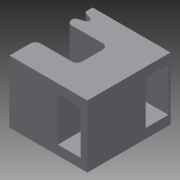
# Autodesk Inventor part: Hook2
Saved by Autodesk Inventor 2015 (Build 190159000, 159)
## iProperties
Created: 2015-01-19
Part Number: Hook2
Material: Generic
Document SubType Name: Modeling
Designer: nilesstanton
Density: 1 g/cm^3
Appearance: Default
Author: nilesstanton
Autodesk Inventor part; units mm, degrees
ref_plane "YZ Plane" through (0, 0, 0) normal (1, 0, 0) x (0, 1, 0)
ref_plane "XZ Plane" through (0, 0, 0) normal (0, 1, 0) x (-1, 0, 0)
ref_plane "XY Plane" through (0, 0, 0) normal (0, 0, 1) x (1, 0, 0)
sketch "Sketch1" plane through (0, 0, 0) normal (0, 1, 0) x (-1, 0, 0)
  line L0 (0, 0) -> (0, 101.6)
  line L1 (44.45, 101.6) -> (0, 101.6)
  line L2 (0, 0) -> (95.25, 0)
  line L3 (44.45, 31.75) -> (95.25, 31.75)
  line L4 (95.25, 31.75) -> (95.25, 22.225)
  line L5 (95.25, 0) -> (95.25, 9.525)
  line L6 (95.25, 22.225) -> (76.2, 15.875)
  line L7 (76.2, 15.875) -> (95.25, 9.525)
  line L8 (44.45, 101.6) -> (95.25, 101.6)
  line L9 (95.25, 101.6) -> (95.25, 69.85)
  line L10 (95.25, 69.85) -> (44.45, 69.85)
  line L11 (44.45, 69.85) -> (44.45, 31.75)
  dimension "d0" = 101.6
  dimension "d1" = 44.45
  dimension "d3" = 95.25
  dimension "d4" = 9.525
  dimension "d5" = 69.85
  dimension "d6" = 19.05
  dimension "d23" = 38.1
  dimension "d24" = 50.8
  constraints: 24 end point, 4 horizontal, 4 vertical, 2 collinear, 2 equal length, 1 parallel, 1 perpendicular
  measures "d0" distance of L0.start L0.end
  measures "d1" distance of L1.start L0.end
  measures "d3" distance of L0.start L2.end
  measures "d4" distance of L2.end L5.end
  measures "d5" distance of L1.start L3.start
  measures "d6" horizontal distance of L4.end L6.end
  measures "d23" distance between parallel lines of L3 L10
  measures "d24" distance of L3.start L3.end
extrude "Extrusion1" add sketch "Sketch1" along normal blind 76.2
fillet "Fillet1" radius 6.35 1 edges at (-95.25, 38.1, 31.75)
fillet "Fillet2" radius 3.175 1 edges at (-76.2, 38.1, 15.875)
fillet "Fillet3" radius 3.175 1 edges at (-95.25, 38.1, 22.225)
fillet "Fillet4" radius 3.175 1 edges at (-95.25, 38.1, 9.525)
sketch "Sketch2" plane through (-44.45, 0, 101.6) normal (0, 0, 1) x (1, 0, 0)
  line L0 (36.195, 11.43) -> (8.255, 11.43)
  line L1 (8.255, 11.43) -> (8.255, 64.77)
  line L2 (8.255, 64.77) -> (36.195, 64.77)
  line L3 (36.195, 64.77) -> (36.195, 11.43)
  line L4 (0, 0) -> (0, 76.2) construction
  line L5 (0, 0) -> (0, 76.2) projected
  line L6 (44.45, 76.2) -> (0, 76.2) construction
  line L7 (44.45, 76.2) -> (-50.8, 76.2) projected
  line L8 (44.45, 76.2) -> (44.45, 0) construction
  line L9 (44.45, 0) -> (44.45, 76.2) projected
  line L10 (44.45, 0) -> (0, 0) construction
  line L11 (-50.8, 0) -> (44.45, 0) projected
  dimension "d14" = 11.43
  dimension "d18" = 11.43
  dimension "d19" = 8.255
  dimension "d20" = 8.255
  constraints: 16 end point, 4 collinear, 2 parallel, 1 horizontal, 1 perpendicular
  measures "d14" distance between parallel lines of L0 L10
  measures "d18" distance between parallel lines of L6 L2
  measures "d19" distance between parallel lines of L4 L1
  measures "d20" distance between parallel lines of L8 L3
extrude "Extrusion2" cut sketch "Sketch2" against normal blind 63.5 contours L0 L1 L2 L3
fillet "Fillet5" radius 6.35 1 edges at (-95.25, 38.1, 69.85)
fillet "Fillet6" radius 6.35 1 edges at (-44.45, 38.1, 31.75)
fillet "Fillet7" radius 6.35 1 edges at (-44.45, 38.1, 69.85)
sketch "Sketch3" plane through (0, 0, 101.6) normal (1, 0, 0) x (0, 0, -1)
  line L0 (99.06, 11.43) -> (71.12, 11.43)
  line L1 (71.12, 11.43) -> (71.12, 64.77)
  line L2 (71.12, 64.77) -> (99.06, 64.77)
  line L3 (99.06, 64.77) -> (99.06, 11.43)
  line L4 (101.6, 0) -> (101.6, 76.2) construction
  line L5 (101.6, 0) -> (101.6, 76.2) projected
  line L6 (101.6, 76.2) -> (0, 76.2) construction
  dimension "d28" = 53.34
  dimension "d29" = 27.94
  dimension "d30" = 2.54
  dimension "d31" = 11.43
  constraints: 12 end point, 3 equal length, 2 perpendicular, 1 horizontal
  measures "d28" distance of L2.end L0.start
  measures "d29" distance of L0.start L0.end
  measures "d30" distance between parallel lines of L4 L3
  measures "d31" distance between parallel lines of L6 L2
extrude "Extrusion3" cut sketch "Sketch3" against normal blind 76.2
body "Solid1"
